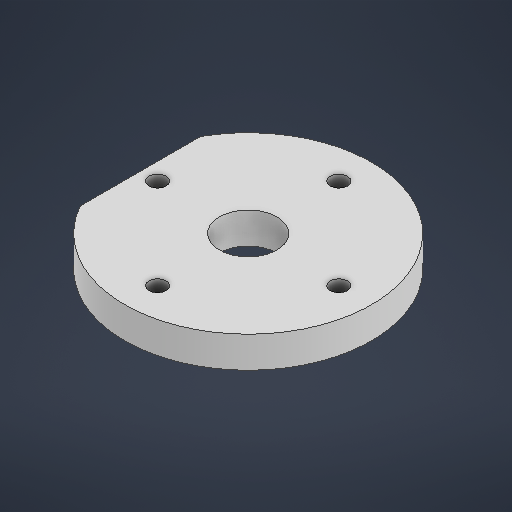
# Autodesk Inventor part: Adapter Plate
Saved by Autodesk Inventor 2025 (Build 290162000, 162)
## iProperties
Created: 2024-09-13
Part Number: Adapter Plate
Material: Generic
Document SubType Name: Modeling
Designer: mayhe
Density: 1 g/cm^3
Appearance: Default
Author: mayhe
Autodesk Inventor part; units mm, degrees
ref_plane "YZ Plane" through (0, 0, 0) normal (1, 0, 0) x (0, 1, 0)
ref_plane "XZ Plane" through (0, 0, 0) normal (0, 1, 0) x (-1, 0, 0)
ref_plane "XY Plane" through (0, 0, 0) normal (0, 0, 1) x (1, 0, 0)
sketch "Sketch1" plane through (0, 0, 0) normal (0, 1, 0) x (-1, 0, 0)
  circle A0 centre (0, 0) radius 39.5
  circle A1 centre (0, 0) radius 10
  circle A2 centre (0, 0) radius 29
  circle A3 centre (29, 0) radius 2.75
  circle A4 centre (0, 29) radius 2.75
  circle A5 centre (-29, 0) radius 2.75
  circle A6 centre (0, -29) radius 2.75
  dimension "d2" = 58
  dimension "d0" = 79
  dimension "d1" = 20
  dimension "d3" = 5.5
  dimension "d6" = 360
  constraints: 6 centre point, 3 coincident, 1 horizontal alignment, 11 other
  measures "d0" diameter of A0
  measures "d1" diameter of A1
  measures "d3" diameter of A3
extrude "Extrusion1" add sketch "Sketch1" along normal blind 10 contours A0 | A1 | A3 A2 A6 A5 A4
sketch "Sketch3" plane through (0, 10, 0) normal (0, 1, 0) x (1, 0, 0)
  line L0 (-34.5, 50.157) -> (-34.5, -49.8555)
  circle A0 centre (0, 0) radius 39.5 projected
  point P0 (-34.5, -19.2354)
  point P1 (-34.5, 19.2354)
  dimension "d18" = 5
  constraints: 2 end point, 1 vertical
  measures "d18" distance edge to line of A0 L0
extrude "Extrusion3" cut sketch "Sketch3" along normal through all both and the other way through all contours L0 A0 picked at (-35.5583, 3.956)
sketch "Sketch4" plane through (0, 0, 0) normal (0, -1, 0) x (1, 0, 0)
  circle A0 centre (0, 0) radius 9.2075
  dimension "d21" = 18.415
  constraints: 1 centre point, 1 coincident
  measures "d21" diameter of A0
extrude "Extrusion4" cut sketch "Sketch4" against normal through all
sketch "Sketch5" plane through (0, 0, 0) normal (0, -1, 0) x (1, 0, 0)
  line L0 (33, -2.3094) -> (29, -4.6188)
  line L1 (29, -4.6188) -> (25, -2.3094)
  line L2 (25, -2.3094) -> (25, 2.3094)
  line L3 (25, 2.3094) -> (29, 4.6188)
  line L4 (29, 4.6188) -> (33, 2.3094)
  line L5 (33, 2.3094) -> (33, -2.3094)
  circle A0 centre (29, 0) radius 2.75
  line L6 (-2.3094, 33) -> (2.3094, 33)
  line L7 (4.6188, 29) -> (2.3094, 25)
  line L8 (2.3094, 25) -> (-2.3094, 25)
  line L9 (-2.3094, 25) -> (-4.6188, 29)
  circle A1 centre (0, 29) radius 2.75
  line L10 (2.3094, 33) -> (4.6188, 29)
  line L11 (-4.6188, 29) -> (-2.3094, 33)
  line L12 (-33, -2.3094) -> (-33, 2.3094)
  line L13 (-29, 4.6188) -> (-25, 2.3094)
  line L14 (-25, 2.3094) -> (-25, -2.3094)
  line L15 (-25, -2.3094) -> (-29, -4.6188)
  circle A2 centre (-29, 0) radius 2.75
  line L16 (-33, 2.3094) -> (-29, 4.6188)
  line L17 (-29, -4.6188) -> (-33, -2.3094)
  line L18 (2.3094, -33) -> (-2.3094, -33)
  line L19 (-4.6188, -29) -> (-2.3094, -25)
  line L20 (-2.3094, -25) -> (2.3094, -25)
  line L21 (2.3094, -25) -> (4.6188, -29)
  circle A3 centre (0, -29) radius 2.75
  line L22 (-2.3094, -33) -> (-4.6188, -29)
  line L23 (4.6188, -29) -> (2.3094, -33)
  point P0 (0, 0)
  point P1 (0, 0)
  point P2 (33, 0)
  point P3 (0, 33)
  point P4 (-33, 0)
  point P5 (0, -33)
  dimension "d27" = 360
  constraints: 48 end point, 4 centre point, 2 coincident, 1 midpoint, 74 other
extrude "Extrusion5" cut sketch "Sketch5" against normal blind 5
body "Solid1"
